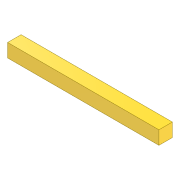
# Autodesk Inventor part: Bone5_4_fix
Saved by Autodesk Inventor 2020 (Build 240168000, 168)
## iProperties
Created: 2021-03-12
Part Number: Bone5_4_fix
Material: Generic
Document SubType Name: Modeling
Designer: deox
Density: 1 g/cm^3
Appearance: Glossy - Gold
Author: deox
Autodesk Inventor part; units mm, degrees
ref_plane "YZ Plane" through (0, 0, 0) normal (1, 0, 0) x (0, 1, 0)
ref_plane "XZ Plane" through (0, 0, 0) normal (0, 1, 0) x (-1, 0, 0)
ref_plane "XY Plane" through (0, 0, 0) normal (0, 0, 1) x (1, 0, 0)
sketch "Sketch1" plane through (0, 0, 0) normal (1, 0, 0) x (0, 1, 0)
  line L0 (-0.1, 0.1) -> (0.1, 0.1)
  line L1 (0.1, 0.1) -> (0.1, -0.1)
  line L2 (0.1, -0.1) -> (-0.1, -0.1)
  line L3 (-0.1, -0.1) -> (-0.1, 0.1)
  line L4 (-0.1, 0.1) -> (0.1, -0.1) construction
  line L5 (0.1, 0.1) -> (-0.1, -0.1) construction
  point P0 (0, 0)
  dimension "d0" = 0.2
  dimension "d1" = 0.2
  constraints: 12 end point, 2 midpoint, 2 parallel, 1 horizontal, 1 perpendicular
  measures "d0" distance of L1.end L2.end
  measures "d1" distance of L0.end L1.end
extrude "Extrusion1" add sketch "Sketch1" against normal mid plane 2.25
body "Solid1"
